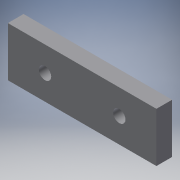
# Autodesk Inventor part: double90
Saved by Autodesk Inventor 2019 (Build 230136000, 136)
## iProperties
Created: 2019-05-07
Part Number: double90
Material: Generic
Document SubType Name: Modeling
Designer: Alex Jones
Density: 1 g/cm^3
Appearance: Default
Author: Alex Jones
Autodesk Inventor part; units mm, degrees
ref_plane "YZ Plane" through (0, 0, 0) normal (1, 0, 0) x (0, 1, 0)
ref_plane "XZ Plane" through (0, 0, 0) normal (0, 1, 0) x (-1, 0, 0)
ref_plane "XY Plane" through (0, 0, 0) normal (0, 0, 1) x (1, 0, 0)
sketch "Sketch1" plane through (0, 0, 0) normal (0, 0, 1) x (1, 0, 0)
  line L0 (0, -1.25) -> (250, -1.25) construction
  line L1 (0, -1.25) -> (0, -6.4) projected
  line L2 (0, -6.4) -> (250, -6.4) construction
  line L3 (250, -1.25) -> (250, -6.4) projected
  line L4 (250, -18.75) -> (0, -18.75) construction
  line L5 (250, -13.6) -> (250, -18.75) projected
  line L6 (0, -13.6) -> (250, -13.6) construction
  line L7 (0, -13.6) -> (0, -18.75) projected
  line L8 (0, -20) -> (250, -20) construction
  line L9 (250, 0) -> (0, 0) construction
  line L10 (24.6484, -20) -> (84.6484, -20)
  line L11 (84.6484, -20) -> (84.6484, 0)
  line L12 (84.6484, 0) -> (24.6484, 0)
  line L13 (24.6484, 0) -> (24.6484, -20)
  line L14 (54.6484, -20) -> (54.6484, 0) construction
  circle A0 centre (67.3484, -10) radius 2.75
  circle A1 centre (41.9484, -10) radius 2.75
  line L15 (54.6484, -10) -> (41.9484, -10) construction
  line L16 (54.6484, -10) -> (67.3484, -10) construction
  point P0 (0, 0)
  dimension "d0" = 60
  dimension "d1" = 5.5
  dimension "d2" = 5.5
  dimension "d11" = 12.7
  constraints: 14 end point, 3 horizontal, 3 midpoint, 2 centre point, 2 parallel, 2 point on line, 1 collinear, 1 perpendicular
  measures "d0" distance between parallel lines of L11 L13
  measures "d1" diameter of A1
  measures "d2" diameter of A0
  measures "d11" distance of L15.start L16.end
extrude "Extrusion1" add sketch "Sketch1" along normal blind 5.08
sketch "Sketch2" plane through (0, 0, 5.08) normal (0, 0, 1) x (1, 0, 0)
  line L0 (84.6484, 0) -> (24.6484, 0) projected
  line L1 (84.6484, -20) -> (84.6484, 0) projected
  line L2 (24.6484, 0) -> (84.6484, 0)
  line L3 (84.6484, 0) -> (84.6484, -5.08)
  line L4 (84.6484, -5.08) -> (24.6484, -5.08)
  line L5 (24.6484, -5.08) -> (24.6484, 0)
  point P0 (0, 0)
  dimension "d5" = 5.08
  constraints: 8 end point, 2 parallel, 1 horizontal, 1 perpendicular, 1 point on line
  measures "d5" distance between parallel lines of L0 L4
extrude "Extrusion2" add sketch "Sketch2" along normal blind 14.92
sketch "Sketch3" plane through (24.6484, -5.08, 5.08) normal (0, -1, 0) x (1, 0, 0)
  line L0 (0, -5.08) -> (0, 14.92) projected
  line L1 (0, 0) -> (60, 0) projected
  line L2 (0, 14.92) -> (0, 0)
  line L3 (60, -5.08) -> (60, 14.92) projected
  line L4 (19.1525, 952.0343) -> (19.1525, -47.9657) construction
  line L5 (19.1525, 952.0343) -> (14.0025, 952.0343) projected
  line L6 (14.0025, 952.0343) -> (14.0025, -47.9657) construction
  line L7 (19.1525, -47.9657) -> (14.0025, -47.9657) projected
  line L8 (1.6525, -47.9657) -> (1.6525, 952.0343) construction
  line L9 (6.8025, -47.9657) -> (1.6525, -47.9657) projected
  line L10 (6.8025, 952.0343) -> (6.8025, -47.9657) construction
  line L11 (6.8025, 952.0343) -> (1.6525, 952.0343) projected
  line L12 (0, 7.46) -> (1.6525, 7.46)
  line L13 (6.8025, 7.46) -> (14.0025, 7.46) construction
  line L14 (41.6525, -47.9657) -> (41.6525, 952.0343) construction
  line L15 (41.6525, -47.9657) -> (46.8025, -47.9657) projected
  line L16 (46.8025, -47.9657) -> (46.8025, 952.0343) construction
  line L17 (41.6525, 952.0343) -> (46.8025, 952.0343) projected
  line L18 (59.1525, 952.0343) -> (59.1525, -47.9657) construction
  line L19 (54.0025, 952.0343) -> (59.1525, 952.0343) projected
  line L20 (54.0025, -47.9657) -> (54.0025, 952.0343) construction
  line L21 (54.0025, -47.9657) -> (59.1525, -47.9657) projected
  line L22 (46.8025, 7.46) -> (54.0025, 7.46) construction
  line L23 (59.1525, 7.46) -> (60, 7.46)
  circle A0 centre (50.4025, 7.46) radius 2.75
  circle A1 centre (10.4025, 7.46) radius 2.75
  point P0 (-24.6484, -5.08)
  dimension "d8" = 5.5
  constraints: 10 end point, 7 point on line, 4 horizontal, 3 midpoint, 2 centre point, 1 equal radius, 1 perpendicular
  measures "d8" diameter of A1
extrude "Extrusion3" cut sketch "Sketch3" against normal blind 14.92
sketch "Sketch4" plane through (84.6484, -20, 0) normal (1, 0, 0) x (0, 0, -1)
  line L0 (-5.08, 0) -> (-5.08, 14.92) projected
  line L1 (-5.08, 14.92) -> (-20, 14.92) projected
  line L2 (-5.08, 0) -> (-20, 14.92)
  line L3 (-20, 14.92) -> (-5.08, 14.92)
  line L4 (-5.08, 14.92) -> (-5.08, 0)
  point P0 (0, 20)
  constraints: 6 end point, 1 collinear, 1 perpendicular
extrude "Extrusion4" add sketch "Sketch4" against normal up to surface (60 mm away)
sketch "Sketch5" plane through (0, 0, 20) normal (0, 0, 1) x (1, 0, 0)
  line L0 (32.3009, 0) -> (37.8009, 0) projected
  line L1 (72.3009, 0) -> (77.8009, 0) projected
  circle A0 centre (41.9484, -10) radius 2.75 projected
  circle A1 centre (67.3484, -10) radius 2.75 projected
  line L2 (84.6484, 0) -> (24.6484, 0) projected
  line L3 (54.6484, 0) -> (54.6484, -20)
  line L4 (24.6484, -20) -> (84.6484, -20) projected
  line L5 (59.7284, -20) -> (49.5684, -20)
  line L6 (49.5684, -20) -> (49.5684, 0)
  line L7 (49.5684, 0) -> (59.7284, 0)
  line L8 (59.7284, 0) -> (59.7284, -20)
  line L9 (59.7284, -20) -> (49.5684, 0) construction
  line L10 (49.5684, -20) -> (59.7284, 0) construction
  line L11 (84.6484, -20) -> (82.1084, -20)
  line L12 (82.1084, -20) -> (82.1084, 0)
  line L13 (82.1084, 0) -> (84.6484, 0)
  line L14 (84.6484, 0) -> (84.6484, -20)
  line L15 (24.6484, -20) -> (27.1884, -20)
  line L16 (27.1884, -20) -> (27.1884, 0)
  line L17 (27.1884, 0) -> (24.6484, 0)
  line L18 (24.6484, 0) -> (24.6484, -20)
  line L19 (24.6484, -5.08) -> (84.6484, -5.08) projected
  line L20 (84.6484, 0) -> (24.6484, 0)
  line L21 (24.6484, 0) -> (24.6484, -5.08)
  line L22 (24.6484, -5.08) -> (84.6484, -5.08)
  line L23 (84.6484, -5.08) -> (84.6484, 0)
  line L24 (59.7284, -20) -> (82.1084, -20)
  line L25 (82.1084, -20) -> (82.1084, -5.08)
  line L26 (82.1084, -5.08) -> (59.7284, -5.08)
  line L27 (59.7284, -5.08) -> (59.7284, -20)
  line L28 (27.1884, -20) -> (49.5684, -20)
  line L29 (49.5684, -20) -> (49.5684, -5.08)
  line L30 (49.5684, -5.08) -> (27.1884, -5.08)
  line L31 (27.1884, -5.08) -> (27.1884, -20)
  point P0 (0, 0)
  point P1 (54.6484, -10)
  dimension "d14" = 2.54
  dimension "d15" = 2.54
  dimension "d16" = 10.16
  constraints: 54 end point, 12 parallel, 6 horizontal, 6 perpendicular, 4 midpoint, 4 point on line, 5 other
  measures "d14" distance between parallel lines of L18 L16
  measures "d15" distance between parallel lines of L14 L12
  measures "d16" distance between parallel lines of L6 L8
extrude "Extrusion5" cut sketch "Sketch5" against normal blind 14.92 contours L19 L6 L4 L16 | L19 L12 L4 L8 | A0 | A1
body "Solid1"
